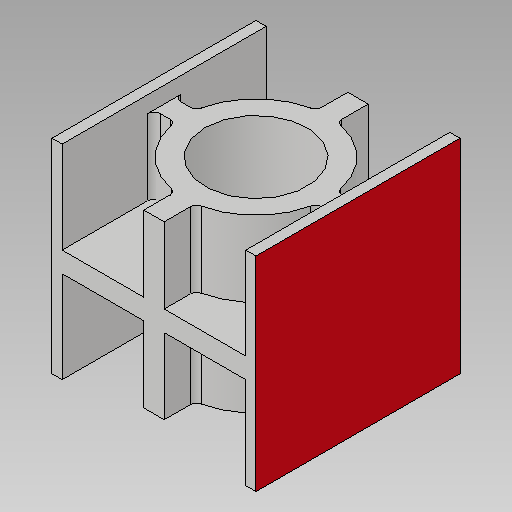
# Autodesk Inventor part: beam_inner_part
Saved by Autodesk Inventor 2020 (Build 240168000, 168)
## iProperties
Created: 2019-04-27
Part Number: beam_inner_part
Material: Generic
Document SubType Name: Modeling
Designer: Varga Daniel
Density: 1 g/cm^3
Appearance: Default
Outer_edge_fillet: 0,100 mm
Author: Varga Daniel
Autodesk Inventor part; units mm, degrees
ref_plane "YZ Plane" through (0, 0, 0) normal (1, 0, 0) x (0, 1, 0)
ref_plane "XZ Plane" through (0, 0, 0) normal (0, 1, 0) x (-1, 0, 0)
ref_plane "XY Plane" through (0, 0, 0) normal (0, 0, 1) x (1, 0, 0)
derived "Base_part.ipt"
sketch "Beam_sketch" plane through (0, 0, 0) normal (0, 1, 0) x (-1, 0, 0)
  circle A0 centre (0, 0) radius 2.5
  line L0 (0, 0) -> (0, -5.5751) construction
  line L1 (3.6649, 0) -> (-4.8297, 0) construction
  arc A1 (-5, 0) -> (0, -5) centre (0, 0) ccw
  line L2 (0, -5) -> (5, -5)
  line L3 (-5, 0) -> (-5, 5)
  line L4 (-5, 5) -> (5, 5)
  line L5 (5, 5) -> (5, -5)
  line L6 (0.5, -3.4641) -> (0.5, -4)
  line L7 (-0.5, -3.2619) -> (-0.5, -4)
  line L8 (0.5, 3.4641) -> (0.5, 4)
  line L9 (-0.5, 3.4641) -> (-0.5, 4)
  line L10 (3.4641, -0.5) -> (4, -0.5)
  line L11 (3.4641, 0.5) -> (4, 0.5)
  line L12 (-3.2619, -0.5) -> (-4, -0.5)
  line L13 (-3.4641, 0.5) -> (-4, 0.5)
  line L14 (-0.5, -4) -> (4, -4)
  arc A2 (-0.5, 3.4641) -> (-3.4641, 0.5) centre (0, 0) ccw
  arc A3 (-3.2619, -0.5) -> (-0.5, -3.2619) centre (0, 0) ccw
  arc A4 (-4.1701, -0.5) -> (-0.5, -4.1701) centre (0, 0) ccw
  line L15 (4, -4) -> (4, -0.5)
  line L16 (4, -0.5) -> (4, 4)
  line L17 (4, 4) -> (0.5, 4)
  line L18 (0.5, 4) -> (-4, 4)
  line L19 (-4, 4) -> (-4, -0.5)
  arc A5 (0.5, -3.4641) -> (3.4641, -0.5) centre (0, 0) ccw
  arc A6 (3.4641, 0.5) -> (0.5, 3.4641) centre (0, 0) ccw
  line L20 (-4, -0.5) -> (-4.1701, -0.5)
  line L21 (-0.5, -4) -> (-0.5, -4.1701)
sketch "Sketch2" plane through (0, 0, 0) normal (0, 1, 0) x (-1, 0, 0)
  line L0 (3.4641, 0.5) -> (4, 0.5) projected
  line L1 (3.4641, -0.5) -> (4, -0.5) projected
  arc A0 (0.5, -3.4641) -> (3.4641, -0.5) centre (0, 0) ccw projected
  circle A1 centre (0, 0) radius 2.5 projected
  arc A2 (3.4641, 0.5) -> (0.5, 3.4641) centre (0, 0) ccw projected
  line L2 (0.5, 3.4641) -> (0.5, 4) projected
  line L3 (0.5, -3.4641) -> (0.5, -4) projected
  line L4 (0, 0) -> (0, -5.5751) construction
  line L5 (3.6649, 0) -> (-4.8297, 0) construction
  line L6 (5, -5) -> (5, 5)
  line L7 (5, 5) -> (4.023, 5)
  line L8 (5, 5) -> (5, 5) construction
  line L9 (5, -5) -> (5, -5) construction
  line L10 (5, -5) -> (0, -5)
  line L11 (0.5, -4) -> (0.5, -5)
  line L12 (4.023, 5) -> (0.023, 5)
  line L13 (0.5, 4) -> (0.5, 5)
  line L14 (-3.4641, 0.5) -> (-4.5, 0.5)
  line L15 (-3.4641, -0.5) -> (-4.5, -0.5)
  arc A3 (-3.4641, -0.5) -> (-0.5, -3.4641) centre (0, 0) ccw
  arc A4 (-0.5, 3.4641) -> (-3.4641, 0.5) centre (0, 0) ccw
  line L16 (-0.5, 3.4641) -> (-0.5, 4)
  line L17 (-0.5, -3.4641) -> (-0.5, -4)
  line L18 (-4, -5) -> (-5, -5)
  line L19 (-5, -5) -> (-5, 5)
  line L20 (-5, 5) -> (-4.023, 5)
  line L21 (-4, -5) -> (0, -5)
  line L22 (-0.5, -4) -> (-0.5, -5)
  line L23 (-4.023, 5) -> (0.023, 5)
  line L24 (-0.5, 4) -> (-0.5, 5)
  line L25 (-4.5, -5) -> (-4.5, 5)
  line L26 (4.5, -5) -> (4.5, 5)
  line L27 (4, 0.5) -> (4.5, 0.5)
  line L28 (4, -0.5) -> (4.5, -0.5)
  point P0 (4, 4)
  point P1 (4, -4)
  point P2 (4, -5)
  point P3 (-4, -0.5)
  point P4 (-4, 0.5)
  point P5 (-3.6649, 0)
  dimension "d9" = 10
  dimension "d11" = 0.5
  dimension "d12" = 10
  dimension "d13" = 0.5
  dimension "d14" = 10
  constraints: 46 end point, 15 point on line, 15 symmetric about line, 4 point on circle, 3 perpendicular, 2 centre point, 2 horizontal, 2 parallel, 1 midpoint, 1 vertical, 2 other
  measures "d9" diameter of L10 L5
  measures "d11" distance between parallel lines of L19 L25
  measures "d12" diameter of L6 L4
  measures "d13" distance between parallel lines of L6 L26
  measures "d14" diameter of L12 L5
extrude "Extrusion1" add sketch "Sketch2" along normal mid plane 10 contours L26 L7 L6 L10 | L25 L18 L19 L20
extrude "Extrusion2" add sketch "Sketch2" along normal mid plane 8.4 contours L0 L27 L26 L28 L1 A0 L3 L11 L10 L21 L22 L17 A3 L15 L25 L14 A4 L16 L24 L23 L12 L13 L2 A2
extrude "Extrusion3" add sketch "Sketch2" along normal mid plane 1 contours A2 L2 L13 L12 L7 L26 L27 L0 | L26 L10 L11 L3 A0 L1 L28 | L24 L16 A4 L14 L25 L20 L23 | L21 L18 L25 L15 A3 L17 L22
fillet "Fillet1" radius 0.3 24 edges at (-0.5, 2.35, 3.4641) (0.5, 2.35, 3.4641) (3.4641, 2.35, 0.5) (-3.4641, 2.35, 0.5) (-0.5, 2.35, -3.4641) (-3.4641, 2.35, -0.5) (0.5, 2.35, -3.4641) (3.4641, 2.35, -0.5) (-0.5, -2.35, -3.4641) (0.5, -2.35, -3.4641) (3.4641, -2.35, -0.5) (-3.4641, -2.35, -0.5) (-0.5, -2.35, 3.4641) (-3.4641, -2.35, 0.5) (0.5, -2.35, 3.4641) (3.4641, -2.35, 0.5) (-4.5, 2.35, -0.5) (-4.5, 2.35, 0.5) (4.5, 2.35, 0.5) (4.5, 2.35, -0.5) (4.5, -2.35, 0.5) (4.5, -2.35, -0.5) (-4.5, -2.35, -0.5) (-4.5, -2.35, 0.5)
equation "\"d9\" = Outer_width"
equation "\"d11\" = 0.5 * Wall_thickness"
equation "\"d12\" = Outer_width"
equation "\"d13\" = 0.5 * Wall_thickness"
equation "\"d14\" = Outer_width"
equation "\"d2\" = Overall_height"
equation "\"d4\" = Hole_height"
equation "\"d6\" = Inner_height"
equation "\"d8\" = Inner_fillet"
equation "\"Outer_width\" = 10"
equation "\"Wall_thickness\" = 1"
equation "\"Overall_height\" = 10"
equation "\"Hole_height\" = 8.4"
equation "\"Inner_height\" = 1"
equation "\"Inner_fillet\" = 0.3"
body "Solid1"
